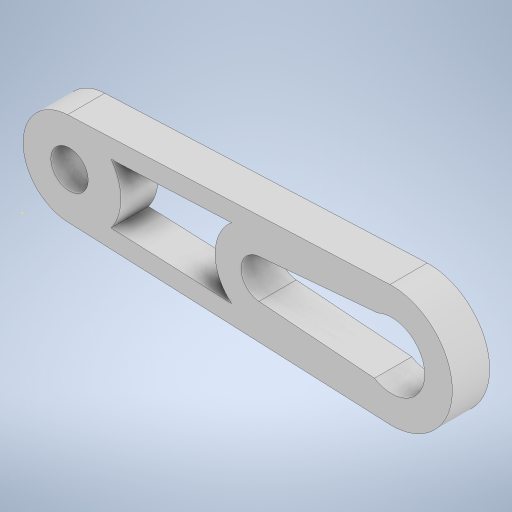
# Autodesk Inventor part: Brazo conductor vertical 2
Saved by Autodesk Inventor 2023 (Build 270158000, 158)
## iProperties
Created: 2023-11-09
Part Number: Brazo conductor vertical 2
Material: Genérico
Description: Model
Document SubType Name: Modeling
Designer: JULIAN
Authority: Unknown
Density: 1 g/cm^3
Appearance: Valor por defecto
Title: Shape Model
Autodesk Inventor part; units mm, degrees
ref_plane "YZ Plane" through (0, 0, 0) normal (1, 0, 0) x (0, 1, 0)
ref_plane "XZ Plane" through (0, 0, 0) normal (0, 1, 0) x (-1, 0, 0)
ref_plane "Plano de trabajo1" through (29.022, 0.5321, 4.5375) normal (0, 0, -1) x (-0.9991, 0.0429, 0)
sketch "Boceto4" plane through (29.022, 0.5321, 4.5375) normal (0, 0, -1) x (-0.9991, 0.0429, 0)
  line L0 (-17.235, 7.0614) -> (-17.2593, 6.4952) projected
  line L1 (-14.4773, 1.1869) -> (-14.926, 1.531) projected
  line L2 (-14.4918, 11.8169) -> (-14.0144, 12.1218) projected
  arc A0 (-9.7469, 12.9526) -> (-9.7469, 12.9526) centre (-10.309, 6.477) ccw
  arc A1 (-8.6792, 9.6202) -> (-8.6041, 3.3739) centre (-10.309, 6.477) ccw
  arc A2 (3.8205, 3.7806) -> (3.9999, 7.9608) centre (3.7273, 5.8786) ccw
  arc A3 (24.2012, 0.0282) -> (24.6354, 9.9665) centre (24.2047, 5.0067) ccw
  circle A4 centre (24.2067, 5.004) radius 1.9965
  arc A5 (-9.8364, 12.9598) -> (-10.3131, -0.023) centre (-10.309, 6.477) ccw
  line L3 (19.8726, 8.3837) -> (19.8889, 8.371) projected
  arc A6 (19.8726, 8.3837) -> (19.6042, 2) centre (24.2067, 5.004) ccw
  arc A7 (22.3471, 10.1759) -> (22.3391, 10.1731) centre (24.2067, 5.004) ccw
  arc A8 (6.6866, 2) -> (7.0079, 9.4895) centre (3.7273, 5.8786) ccw
  line L4 (-9.8364, 12.9598) -> (24.6354, 9.9665)
  line L5 (-8.6792, 9.6202) -> (3.9999, 7.9608)
  line L6 (-10.3131, -0.023) -> (24.2012, 0.0282)
  line L7 (3.8205, 3.7806) -> (-8.6041, 3.3739)
  line L8 (7.0079, 9.4895) -> (19.8889, 8.371)
  line L9 (19.6042, 2) -> (6.6866, 2)
  point P0 (28.9725, -1.7754)
  point P1 (-10.2027, 12.9761)
  point P2 (24.6399, 6.9529)
  point P3 (19.8643, 8.3731)
  constraints: 18 point on circle, 12 end point, 8 centre point, 4 coincident, 1 horizontal, 1 parallel, 1 tangent, 3 other
extrude "Extrusión3" add sketch "Boceto4" along normal blind 4 contours A0 L5 A1 L7 | L4 A3 L6 A0 L7 A2 L5 picked at (-6.02, 9.6518)
sketch "Boceto5" plane through (29.022, 0.5321, 4.5375) normal (0, 0, 1) x (0.9991, -0.0429, 0)
  point P0 (-28.9725, -1.7754)
